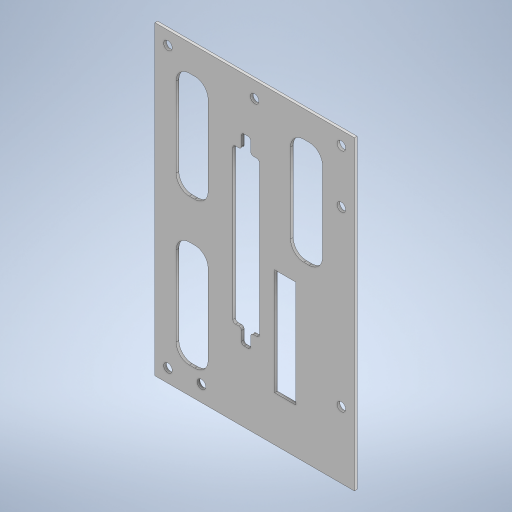
# Autodesk Inventor part: back
Saved by Autodesk Inventor 2023 (Build 270158000, 158)
## iProperties
Created: 2023-05-25
Part Number: back
Material: Generic
Document SubType Name: Sheet Metal
Designer: 310611102
Density: 1 g/cm^3
Sheet Metal Rule: 1mm
Appearance: Default
Author: 310611102
Autodesk Inventor part; units mm, degrees
ref_plane "YZ Plane" through (0, 0, 0) normal (1, 0, 0) x (0, 1, 0)
ref_plane "XZ Plane" through (0, 0, 0) normal (0, 1, 0) x (-1, 0, 0)
ref_plane "XY Plane" through (0, 0, 0) normal (0, 0, 1) x (1, 0, 0)
sketch "Sketch1" plane through (0, 0, 0) normal (0, 0, 1) x (1, 0, 0)
  line L0 (-37.5, 57.5) -> (37.5, 57.5)
  line L1 (37.5, 57.5) -> (37.5, -57.5)
  line L2 (37.5, -57.5) -> (-37.5, -57.5)
  line L3 (-37.5, -57.5) -> (-37.5, 57.5)
  line L4 (-37.5, 57.5) -> (37.5, -57.5) construction
  line L5 (37.5, 57.5) -> (-37.5, -57.5) construction
  line L6 (1.8, 31.5) -> (1.8, -24.5)
  line L7 (-8.2, -24.5) -> (-8.2, 31.5)
  line L8 (-8.2, 32.5) -> (1.8, -25.5) construction
  line L9 (1.8, 32.5) -> (-8.2, -25.5) construction
  line L10 (-3.95, 38) -> (-2.45, 38)
  line L11 (-1.45, 37) -> (-1.45, 33.5)
  line L12 (-4.95, 33.5) -> (-4.95, 37)
  line L13 (-4.95, 38) -> (-1.45, 32.5) construction
  line L14 (-1.45, 38) -> (-4.95, 32.5) construction
  line L15 (-3.95, -31) -> (-2.45, -31)
  line L16 (-1.45, -30) -> (-1.45, -26.5)
  line L17 (-4.95, -26.5) -> (-4.95, -30)
  line L18 (-4.95, -31) -> (-1.45, -25.5) construction
  line L19 (-1.45, -31) -> (-4.95, -25.5) construction
  circle A0 centre (-32.6, 52.5) radius 1.6
  line L20 (0, 0) -> (0, 3.4669)
  line L21 (0, 0) -> (3.1568, 0)
  circle A1 centre (32.6, 52.5) radius 1.6
  circle A2 centre (-32.6, -52.5) radius 1.6
  circle A3 centre (-20, -51.5) radius 1.6
  circle A4 centre (32.6, -32.5) radius 1.6
  circle A5 centre (32.6, 32.5) radius 1.6
  circle A6 centre (0, 51.5) radius 1.6
  line L22 (7.5, -0.5) -> (15.5, -0.5)
  line L23 (15.5, -0.5) -> (15.5, -40.5)
  line L24 (15.5, -40.5) -> (7.5, -40.5)
  line L25 (7.5, -40.5) -> (7.5, -0.5)
  line L26 (7.5, -0.5) -> (15.5, -40.5) construction
  line L27 (15.5, -0.5) -> (7.5, -40.5) construction
  line L28 (-24.5, 47.5) -> (-22.5, 47.5)
  line L29 (-17.5, 42.5) -> (-17.5, 12.5)
  line L30 (-22.5, 7.5) -> (-24.5, 7.5)
  line L31 (-29.5, 12.5) -> (-29.5, 42.5)
  line L32 (-29.5, 47.5) -> (-17.5, 7.5) construction
  line L33 (-17.5, 47.5) -> (-29.5, 7.5) construction
  arc A7 (-24.5, 47.5) -> (-29.5, 42.5) centre (-24.5, 42.5) ccw
  arc A8 (-17.5, 42.5) -> (-22.5, 47.5) centre (-22.5, 42.5) ccw
  arc A9 (-22.5, 7.5) -> (-17.5, 12.5) centre (-22.5, 12.5) ccw
  arc A10 (-29.5, 12.5) -> (-24.5, 7.5) centre (-24.5, 12.5) ccw
  line L34 (-24.5, -47.5) -> (-22.5, -47.5)
  line L35 (-17.5, -42.5) -> (-17.5, -12.5)
  line L36 (-22.5, -7.5) -> (-24.5, -7.5)
  line L37 (-29.5, -12.5) -> (-29.5, -42.5)
  line L38 (-29.5, -47.5) -> (-17.5, -7.5) construction
  line L39 (-17.5, -47.5) -> (-29.5, -7.5) construction
  arc A11 (-29.5, -42.5) -> (-24.5, -47.5) centre (-24.5, -42.5) ccw
  arc A12 (-22.5, -47.5) -> (-17.5, -42.5) centre (-22.5, -42.5) ccw
  arc A13 (-17.5, -12.5) -> (-22.5, -7.5) centre (-22.5, -12.5) ccw
  arc A14 (-24.5, -7.5) -> (-29.5, -12.5) centre (-24.5, -12.5) ccw
  line L40 (18.5, 47.5) -> (20.5, 47.5)
  line L41 (25.5, 42.5) -> (25.5, 12.5)
  line L42 (20.5, 7.5) -> (18.5, 7.5)
  line L43 (13.5, 12.5) -> (13.5, 42.5)
  line L44 (13.5, 47.5) -> (25.5, 7.5) construction
  line L45 (25.5, 47.5) -> (13.5, 7.5) construction
  arc A15 (18.5, 47.5) -> (13.5, 42.5) centre (18.5, 42.5) ccw
  arc A16 (25.5, 42.5) -> (20.5, 47.5) centre (20.5, 42.5) ccw
  arc A17 (20.5, 7.5) -> (25.5, 12.5) centre (20.5, 12.5) ccw
  arc A18 (13.5, 12.5) -> (18.5, 7.5) centre (18.5, 12.5) ccw
  arc A19 (-3.95, 38) -> (-4.95, 37) centre (-3.95, 37) ccw
  arc A20 (-1.45, 37) -> (-2.45, 38) centre (-2.45, 37) ccw
  arc A21 (-4.95, -30) -> (-3.95, -31) centre (-3.95, -30) ccw
  arc A22 (-2.45, -31) -> (-1.45, -30) centre (-2.45, -30) ccw
  line L46 (0.8, -25.5) -> (-0.45, -25.5)
  line L47 (-5.95, -25.5) -> (-7.2, -25.5)
  line L48 (-7.2, 32.5) -> (-5.95, 32.5)
  line L49 (-0.45, 32.5) -> (0.8, 32.5)
  arc A23 (-7.2, 32.5) -> (-8.2, 31.5) centre (-7.2, 31.5) ccw
  arc A24 (-5.95, 32.5) -> (-4.95, 33.5) centre (-5.95, 33.5) ccw
  arc A25 (-1.45, 33.5) -> (-0.45, 32.5) centre (-0.45, 33.5) ccw
  arc A26 (1.8, 31.5) -> (0.8, 32.5) centre (0.8, 31.5) ccw
  arc A27 (0.8, -25.5) -> (1.8, -24.5) centre (0.8, -24.5) ccw
  arc A28 (-0.45, -25.5) -> (-1.45, -26.5) centre (-0.45, -26.5) ccw
  arc A29 (-4.95, -26.5) -> (-5.95, -25.5) centre (-5.95, -26.5) ccw
  arc A30 (-8.2, -24.5) -> (-7.2, -25.5) centre (-7.2, -24.5) ccw
  point P0 (-3.2, 3.5)
  point P1 (-3.2, 35.25)
  point P2 (-3.2, -28.25)
  point P3 (11.5, -20.5)
  point P4 (-23.5, 27.5)
  point P5 (-23.5, -27.5)
  point P6 (19.5, 27.5)
  point P7 (0, -57.5)
  point P8 (0, 57.5)
  dimension "d0" = 75
  dimension "d1" = 115
  dimension "d2" = 3.5
  dimension "d3" = 5.5
  dimension "d4" = 10
  dimension "d5" = 58
  dimension "d6" = 35.7
  dimension "d9" = 3.2
  dimension "d10" = 5
  dimension "d11" = 4.9
  dimension "d14" = 3.2
  dimension "d15" = 6
  dimension "d16" = 3.2
  dimension "d18" = 4.9
  dimension "d19" = 25
  dimension "d20" = 8
  dimension "d21" = 40
  dimension "d23" = 22
  dimension "d24" = 17
  dimension "d25" = 12
  dimension "d26" = 40
  dimension "d27" = 5
  dimension "d28" = 10
  dimension "d29" = 8
  dimension "d30" = 40
  dimension "d31" = 12
  dimension "d32" = 12
  dimension "d33" = 10
  dimension "d34" = 5
  dimension "d36" = 20
  dimension "d37" = 6
  dimension "d38" = 0
  dimension "d39" = 3.2
  dimension "d40" = 1
  dimension "d41" = 25
  dimension "d42" = 1
  measures "d0" distance of L0.start L0.end
  measures "d1" distance of L0.end L1.end
  measures "d2" distance of L13.start L14.start
  measures "d3" distance of L14.start L13.end
  measures "d4" distance of L8.start L9.start
  measures "d5" distance of L9.end L8.start
  measures "d6" distance between parallel lines of L1 L6
  measures "d9" diameter of A0
  measures "d10" distance from line of L0 A0.centre
  measures "d11" distance from line of A0.centre L3
  measures "d14" diameter of A3
  measures "d15" distance from line of L2 A3.centre
  measures "d16" diameter of A4
  measures "d18" distance from line of L1 A4.centre
  measures "d19" distance from line of L2 A4.centre
  measures "d20" distance of L22.start L22.end
  measures "d21" distance of L22.end L23.end
  measures "d23" distance between parallel lines of L1 L23
  measures "d24" distance between parallel lines of L2 L24
  measures "d25" distance of L32.start L33.start
  measures "d26" distance of L33.end L32.start
  measures "d27" radius of A7
  measures "d28" distance between parallel lines of L0 L28
  measures "d29" distance between parallel lines of L3 L31
  measures "d30" distance between parallel lines of L42 L40
  measures "d31" distance of L44.end L45.end
  measures "d32" distance between parallel lines of L1 L41
  measures "d33" distance between parallel lines of L0 L40
  measures "d34" radius of A15
  measures "d36" horizontal distance of point (0, -57.5) A3.centre
  measures "d37" distance from line of L0 A6.centre
  measures "d38" horizontal distance of point (0, 57.5) A6.centre
  measures "d39" diameter of A6
  measures "d40" radius of A19
  measures "d41" distance between parallel lines of L0 L48
  measures "d42" radius of A23
extrude "Plate1" add sketch "Sketch1" along normal blind 1
equation "\"d8\" = 厚度"
equation "\"折彎半徑\" = 厚度"
equation "\"折彎離隙寬度\" = 厚度"
equation "\"折彎離隙深度\" = 0.5 * 厚度"
equation "\"轉角離隙大小\" = 4 * 厚度"
equation "\"最小剩餘\" = 2 * 厚度"
equation "\"轉移半徑\" = 折彎半徑"
equation "\"Jacobi半徑大小\" = 折彎半徑"
equation "\"間隙大小\" = 厚度"
equation "\"厚度\" = 1"
body "Solid1"
